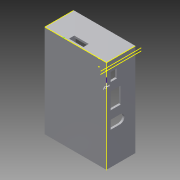
# Autodesk Inventor part: PI_Skal
Saved by Autodesk Inventor 2015 (Build 190159000, 159)
## iProperties
Created: 2015-11-29
Part Number: PI_Skal
Material: Generic
Document SubType Name: Modeling
Designer: abberik
Density: 1 g/cm^3
Appearance: Default
Author: abberik
Autodesk Inventor part; units mm, degrees
sketch "Sketch1" plane through (0, 0, 0) normal (0, 1, 0) x (-1, 0, 0)
  point P0 (0, 0)
sketch "Sketch2" plane through (0, 0, 0) normal (0, 1, 0) x (-1, 0, 0)
  circle A0 centre (0, 0) radius 1.25
  line L0 (60.55, 0) -> (-11.55, 0) projected
  line L1 (0, -71.35) -> (0, 13.35) projected
  circle A1 centre (49, 0) radius 1.25
  circle A2 centre (0, -58) radius 1.25
  circle A3 centre (49, -58) radius 1.25
  dimension "d0" = 2.5
  dimension "d3" = 49
  dimension "d6" = 58
  constraints: 4 centre point, 1 coincident, 1 horizontal, 1 vertical, 6 other
  measures "d0" diameter of A0
  measures "d3" distance of A0.centre A1.centre
  measures "d6" distance of A0.centre A2.centre
extrude "Extrusion1" add sketch "Sketch2" along normal blind 10
sketch "Sketch3" plane through (0, 0, 0) normal (0, 1, 0) x (-1, 0, 0)
  line L0 (52.5, 3.5) -> (-3.5, 3.5)
  line L1 (-3.5, 3.5) -> (-3.5, -85)
  line L2 (-3.5, -85) -> (52.5, -85)
  line L3 (52.5, -85) -> (52.5, 3.5)
  circle A0 centre (49, 0) radius 1.25 projected
  circle A1 centre (49, -58) radius 1.25 projected
  circle A2 centre (0, 0) radius 1.25 projected
  circle A3 centre (0, -58) radius 1.25 projected
  line L4 (54.5, 5.5) -> (-5.5, 5.5)
  line L5 (-5.5, 5.5) -> (-5.5, -87)
  line L6 (-5.5, -87) -> (54.5, -87)
  line L7 (54.5, -87) -> (54.5, 5.5)
  dimension "d11" = 3.5
  dimension "d12" = 27
  dimension "d13" = 3.5
  dimension "d14" = 3.5
  dimension "d15" = 2
  constraints: 16 end point, 4 parallel, 2 perpendicular, 1 horizontal, 3 other
  measures "d11" distance from line of L0 A0.centre
  measures "d12" distance from line of L2 A1.centre
  measures "d13" distance from line of L3 A0.centre
  measures "d14" distance from line of L1 A2.centre
  measures "d15" distance between parallel lines of L1 L5
extrude "Extrusion2" add sketch "Sketch3" along normal blind 2 contours L3 L2 L1 L0 | L7 L6 L5 L4
sketch "Sketch5" plane through (0, 0, 0) normal (0, 0, 1) x (1, 0, 0)
  line L0 (-54.5, 0) -> (5.5, 0) projected
  line L1 (5.5, 0) -> (5.5, 2) projected
  line L2 (-54.5, 2) -> (5.5, 2) projected
  line L3 (-54.5, 0) -> (-54.5, 2) projected
  line L4 (5.5, 0) -> (7.5, 0)
  line L5 (7.5, 0) -> (7.5, 30)
  line L6 (7.5, 30) -> (5.5, 30)
  line L7 (5.5, 30) -> (5.5, 0)
  point P0 (0, 0)
  dimension "d18" = 2
  dimension "d19" = 30
  constraints: 8 end point, 2 parallel, 1 horizontal, 1 perpendicular
  measures "d18" distance of L5.end L6.end
  measures "d19" distance of L4.end L5.end
sketch3d "3D Sketch1"
sketch3d "3D Sketch2"
  line L0 (5.5, 2, -87) -> (5.5, 2, 5.5)
  line L1 (5.5, 2, 5.5) -> (-54.5, 2, 5.5)
  line L2 (-54.5, 2, 5.5) -> (-54.5, 2, -87)
sweep "Sweep2" add profiles "Sketch5" path "3D Sketch2" contours L1 L7 L6 L5 L4
sketch "Sketch6" plane through (7.5, 0, -87) normal (0, 0, -1) x (-1, 0, 0)
  line L0 (2, 30) -> (62, 30)
  line L1 (2, 30) -> (2, 2) projected
  line L2 (2, 25) -> (62, 25)
  line L3 (62, 30) -> (62, 2) projected
  line L4 (2, 25) -> (2, 2)
  line L5 (2, 2) -> (62, 2)
  line L6 (2, 2) -> (62, 2) projected
  line L7 (62, 25) -> (62, 2)
  line L8 (0, 0) -> (0, 30) projected
  line L9 (0, 30) -> (2, 30) projected
  line L10 (64, 0) -> (0, 0) projected
  line L11 (64, 0) -> (64, 30) projected
  line L12 (64, 30) -> (62, 30) projected
  point P0 (7.5, 0)
  dimension "d25" = 5
  constraints: 10 end point, 2 collinear, 2 horizontal, 2 point on line, 1 vertical
  measures "d25" distance between parallel lines of L2 L0
extrude "Extrusion3" add sketch "Sketch6" along normal blind 2 contours L0 L3 L2 L1 | L1 L5 L3 L12 L11 L10 L8 L9
sketch "Sketch8" plane through (-56.5, 30, 7.5) normal (0, 0, 1) x (1, 0, 0)
  line L0 (64, -30) -> (0, -30) projected
  line L1 (0, -30) -> (0, 0) projected
  line L2 (64, -30) -> (64, 0) projected
  point P0 (56.5, -30)
  point P1 (20, -30)
  constraints: 1 point on line
sketch "Sketch9" plane through (0, 2, 0) normal (0, 1, 0) x (1, 0, 0)
  circle A0 centre (0, 0) radius 1.25 projected
  circle A1 centre (0, 0) radius 1.25 projected
  circle A2 centre (-49, 0) radius 1.25 projected
  circle A3 centre (-49, 0) radius 1.25 projected
  circle A4 centre (-49, 58) radius 1.25 projected
  circle A5 centre (-49, 58) radius 1.25 projected
  circle A6 centre (0, 58) radius 1.25 projected
  circle A7 centre (0, 58) radius 1.25 projected
  circle A8 centre (0, 58) radius 1.25 projected
  circle A9 centre (0, 0) radius 2.5
  circle A10 centre (-49, 0) radius 1.25 projected
  circle A11 centre (-49, 0) radius 2.5
  circle A12 centre (0, 58) radius 2.5
  circle A13 centre (-49, 58) radius 2.5
  dimension "d44" = 5
  dimension "d45" = 5
  dimension "d46" = 5
  dimension "d47" = 5
  constraints: 4 centre point, 4 coincident
  measures "d44" diameter of A9
  measures "d45" diameter of A11
  measures "d46" diameter of A12
  measures "d47" diameter of A13
extrude "Extrusion6" add sketch "Sketch9" along normal blind 4
sketch "Sketch11" plane through (7.5, 0, 7.5) normal (1, 0, 0) x (0, 0, -1)
  line L0 (7.5, -6) -> (7.5, 36) projected
  point P0 (7.5, 0)
ref_plane "Work Plane1" through (0, 2, 2.5) normal (0, 0, 1) x (1, 0, 0)
ref_plane "Work Plane2" through (0, 2, 2.8) normal (0, 0, 1) x (1, 0, 0)
sketch "Sketch12" plane through (7.5, 0, 7.5) normal (1, 0, 0) x (0, 0, -1)
  line L0 (7.5, -6) -> (7.5, 36) projected
  line L1 (4.7, -6) -> (4.7, 36) projected
  line L2 (13.1008, 0) -> (18.181, 0)
  line L3 (96.5, 0) -> (0, 0) projected
  point P0 (7.5, 0)
  dimension "d51" = 0
  constraints: 2 end point, 1 horizontal
  measures "d51" distance between parallel lines of L3 L2
ref_plane "Work Plane3" through (-49, 6, -58) normal (0, 1, 0) x (1, 0, 0)
sketch "Sketch13" plane through (7.5, 0, 7.5) normal (1, 0, 0) x (0, 0, -1)
  line L0 (-19.3, 6) -> (115.8, 6) projected
  line L1 (10.8, 4.5) -> (19.8, 4.5)
  line L2 (19.8, 4.5) -> (19.8, 11)
  line L3 (19.8, 11) -> (10.8, 11)
  line L4 (10.8, 11) -> (10.8, 4.5)
  line L5 (28.2, 4.5) -> (45.2, 4.5)
  line L6 (45.2, 4.5) -> (45.2, 15)
  line L7 (45.2, 15) -> (28.2, 15)
  line L8 (28.2, 15) -> (28.2, 4.5)
  line L9 (4.7, -6) -> (4.7, 36) projected
  line L10 (53.7, 4.5) -> (62.7, 4.5)
  line L11 (62.7, 4.5) -> (62.7, 14.1644)
  line L12 (53.7, 14.1644) -> (53.7, 4.5)
  arc A0 (62.7, 14.1644) -> (53.7, 14.1644) centre (58.2, 14.1644) ccw
  point P0 (7.5, 0)
  point P1 (15.3, 11)
  point P2 (36.7, 15)
  dimension "d54" = 1.5
  dimension "d55" = 9
  dimension "d57" = 10.6
  dimension "d58" = 32
  dimension "d60" = 17
  dimension "d61" = 1.5
  dimension "d63" = 9
  dimension "d64" = 53.5
  dimension "d65" = 1.5
  dimension "d66" = 9
  dimension "d67" = 5
  constraints: 22 end point, 5 parallel, 3 horizontal, 3 perpendicular, 2 midpoint, 2 point on circle, 1 centre point
  measures "d54" distance between parallel lines of L1 L0
  measures "d55" distance between parallel lines of L4 L2
  measures "d57" distance from line of L9 point (15.3, 11)
  measures "d58" distance from line of point (36.7, 15) L9
  measures "d60" distance between parallel lines of L6 L8
  measures "d61" distance between parallel lines of L0 L5
  measures "d63" distance between parallel lines of L11 L12
  measures "d64" distance from line of L9 A0.centre
  measures "d65" distance between parallel lines of L0 L10
  measures "d66" distance between parallel lines of L0 L7
  measures "d67" distance between parallel lines of L0 L3
extrude "Extrusion7" cut sketch "Sketch13" against normal up to surface (2 mm away)
ref_plane "Work Plane5" through (2.7, 2, 0) normal (-1, 0, 0) x (0, -1, 0)
ref_plane "Work Plane4" through (2.5, 2, 0) normal (-1, 0, 0) x (0, -1, 0)
sketch "Sketch15" plane through (-56.5, 30, 7.5) normal (0, 0, 1) x (1, 0, 0)
  line L0 (59.2, -36) -> (59.2, 6) projected
  line L1 (-12.8, -24) -> (76.8, -24) projected
  line L2 (23.2, -22.5) -> (38.2, -22.5)
  line L3 (38.2, -22.5) -> (38.2, -28)
  line L4 (38.2, -28) -> (23.2, -28)
  line L5 (23.2, -28) -> (23.2, -22.5)
  point P0 (56.5, -30)
  dimension "d71" = 21
  dimension "d72" = 36
  dimension "d73" = 4
  dimension "d74" = 1.5
  constraints: 8 end point, 2 parallel, 1 horizontal, 1 perpendicular
  measures "d71" distance between parallel lines of L0 L3
  measures "d72" distance between parallel lines of L0 L5
  measures "d73" distance between parallel lines of L4 L1
  measures "d74" distance between parallel lines of L2 L1
extrude "Extrusion8" cut sketch "Sketch15" against normal up to surface (2 mm away)
body "Solid1"
